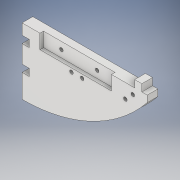
# Autodesk Inventor part: CP003
Saved by Autodesk Inventor 2017 SP1 (Build 210196100, 196)
## iProperties
Created: 2017-05-15
Part Number: CP003
Material: ABS Plastic
Document SubType Name: Modeling
Designer: zallen
Density: 1.06 g/cm^3
Appearance: Smooth - White
Mass: 174.081 g
Surface Area: 322.497 cm^2
Volume: 164.227 cm^3
Author: zallen
Autodesk Inventor part; units mm, degrees
ref_plane "YZ Plane" through (0, 0, 0) normal (1, 0, 0) x (0, 1, 0)
ref_plane "XZ Plane" through (0, 0, 0) normal (0, 1, 0) x (-1, 0, 0)
ref_plane "XY Plane" through (0, 0, 0) normal (0, 0, 1) x (1, 0, 0)
sketch "Sketch1" plane through (0, 0, 0) normal (0, 0, 1) x (1, 0, 0)
  circle A0 centre (0, 132.2876) radius 225 construction
  circle A1 centre (0, 132.2876) radius 200 construction
  line L0 (150, 132.2876) -> (150, 0) construction
  line L1 (150, 0) -> (0, 0)
  line L2 (0, 0) -> (0, -92.7124)
  arc A2 (0, -92.7124) -> (175, -9.1338) centre (0, 132.2876) ccw
  line L3 (157.5, 0) -> (157.5, 10)
  line L4 (157.5, 10) -> (167.5, 10)
  line L5 (167.5, 10) -> (167.5, 0)
  line L6 (150, 0) -> (157.5, 0)
  line L7 (175, -35.9935) -> (175, -9.1338) construction
  line L8 (175, 0) -> (175, -9.1338)
  line L9 (167.5, 0) -> (175, 0)
  line L10 (0, 132.2876) -> (0, -92.7124) construction
  line L11 (0, 132.2876) -> (225, 132.2876) construction
  line L12 (0, 0) -> (130.6185, 0) construction
  dimension "d0" = 450
  dimension "d1" = 25
  dimension "d3" = 10
  dimension "d4" = 10
  dimension "d6" = 7.5
  dimension "d7" = 90
  dimension "d9" = 25
  dimension "d12" = 90
  dimension "d13" = 75
  dimension "d14" = 90
  constraints: 26 end point, 6 point on circle, 5 point on line, 4 perpendicular, 3 horizontal, 2 centre point, 1 coincident, 1 collinear, 1 concentric, 1 parallel, 3 other
  measures "d0" diameter of A0
  measures "d3" distance of L3.start L3.end
  measures "d4" distance of L3.end L4.end
  measures "d6" distance of L0.end L3.start
  measures "d7" angle of L5 L4
  measures "d9" distance between parallel lines of L7 L0
  measures "d12" angle of L10 L11
  measures "d13" distance of L11.end L0.start
  measures "d14" angle of L1 L0
extrude "Extrusion1" add sketch "Sketch1" along normal blind 15
sketch "Sketch2" plane through (0, 0, 15) normal (0, 0, 1) x (1, 0, 0)
  line L0 (0, 0) -> (0, -92.7124) projected
  line L1 (0, -15) -> (10, -15)
  line L2 (10, -15) -> (10, -25)
  line L3 (10, -25) -> (0, -25)
  line L4 (0, -25) -> (0, -15)
  line L5 (0, -50) -> (10, -50)
  line L6 (10, -50) -> (10, -60)
  line L7 (10, -60) -> (0, -60)
  line L8 (0, -60) -> (0, -50)
  line L9 (157.5, 0) -> (0, 0) projected
  dimension "d15" = 10
  dimension "d16" = 10
  dimension "d17" = 10
  dimension "d18" = 10
  dimension "d19" = 25
  dimension "d20" = 15
  constraints: 16 end point, 4 parallel, 2 horizontal, 2 perpendicular, 2 point on line
  measures "d15" distance of L2.end L3.end
  measures "d16" distance of L1.end L2.end
  measures "d17" distance of L6.end L7.end
  measures "d18" distance of L5.end L6.end
  measures "d19" distance between parallel lines of L5 L3
  measures "d20" distance between parallel lines of L1 L9
extrude "Extrusion2" cut sketch "Sketch2" against normal blind 15
sketch "Sketch3" plane through (0, 0, 15) normal (0, 0, 1) x (1, 0, 0)
  line L0 (157.5, 0) -> (0, 0) construction
  line L1 (25, 0) -> (125, 0) construction
  line L2 (125, 0) -> (125, -20) construction
  line L3 (125, -20) -> (25, -20) construction
  line L4 (25, -20) -> (25, 0) construction
  circle A0 centre (50, -10) radius 2.5
  circle A1 centre (100, -10) radius 2.5
  dimension "d23" = 100
  dimension "d24" = 20
  dimension "d25" = 25
  dimension "d26" = 5
  dimension "d27" = 5
  dimension "d28" = 25
  dimension "d29" = 25
  constraints: 8 end point, 2 centre point, 2 parallel, 1 horizontal, 1 perpendicular, 1 point on line
  measures "d23" distance of L2.end L3.end
  measures "d24" distance of L1.end L2.end
  measures "d25" distance from line of L0.end L4
  measures "d26" diameter of A0
  measures "d27" diameter of A1
  measures "d28" distance from line of L4 A0.centre
  measures "d29" distance from line of L2 A1.centre
extrude "Extrusion3" cut sketch "Sketch3" against normal through all
thread "Thread1" size "M5x0.8" class "6H" standard "ANSI Metric M Profile" full length
thread "Thread2" size "M5x0.8" class "6H" standard "ANSI Metric M Profile" full length
sketch "Sketch4" plane through (0, 0, 15) normal (0, 0, 1) x (1, 0, 0)
  line L0 (157.5, 0) -> (0, 0) projected
  line L1 (25, 0) -> (125, 0)
  line L2 (125, 0) -> (125, -20)
  line L3 (125, -20) -> (25, -20)
  line L4 (25, -20) -> (25, 0)
  dimension "d36" = 100
  dimension "d37" = 20
  dimension "d38" = 25
  constraints: 8 end point, 2 parallel, 1 horizontal, 1 perpendicular, 1 point on line
  measures "d36" distance of L2.end L3.end
  measures "d37" distance of L1.end L2.end
  measures "d38" distance from line of L0.end L4
extrude "Extrusion4" cut sketch "Sketch4" against normal blind 5
sketch "Sketch5" plane through (0, 0, 15) normal (0, 0, 1) x (1, 0, 0)
  circle A0 centre (0, 132.2876) radius 225 construction
  arc A1 (0, -92.7124) -> (175, -9.1338) centre (0, 132.2876) ccw construction
  circle A2 centre (0, 132.2876) radius 210 construction
  circle A3 centre (144.4906, -20.1016) radius 2.5
  circle A4 centre (155, -9.3987) radius 2.5
  line L0 (175, -9.1338) -> (175, 0) projected
  point P0 (0, 0)
  dimension "d41" = 450
  dimension "d42" = 15
  dimension "d43" = 5
  dimension "d44" = 5
  dimension "d45" = 15
  dimension "d46" = 20
  constraints: 4 centre point, 2 point on circle, 1 concentric
  measures "d41" diameter of A0
  measures "d42" radial gap between concentric circles of A0 A2
  measures "d43" diameter of A3
  measures "d44" diameter of A4
  measures "d45" distance of A4.centre A3.centre
  measures "d46" distance from line of L0 A4.centre
extrude "Extrusion5" cut sketch "Sketch5" against normal through all
thread "Thread3" size "M5x0.8" class "6H" standard "ANSI Metric M Profile" full length
thread "Thread4" size "M5x0.8" class "6H" standard "ANSI Metric M Profile" full length
sketch "Sketch6" plane through (0, 0, 15) normal (0, 0, 1) x (1, 0, 0)
  circle A0 centre (69.0912, -25.1338) radius 2.5
  circle A1 centre (84.0912, -25.1338) radius 2.5
  line L0 (25, 0) -> (125, 0) projected
  arc A2 (0, -92.7124) -> (175, -9.1338) centre (0, 132.2876) ccw construction
  line L1 (175, -9.1338) -> (-10.7224, -9.1338) construction
  line L2 (0, 0) -> (0, -15) construction
  dimension "d53" = 5
  dimension "d54" = 5
  dimension "d56" = 16
  dimension "d57" = 69.0912
  dimension "d58" = 15
  constraints: 2 centre point, 2 end point, 1 horizontal alignment, 1 perpendicular
  measures "d53" diameter of A0
  measures "d54" diameter of A1
  measures "d56" distance from line of A0.centre L1
  measures "d57" distance from line of L2 A0.centre
  measures "d58" distance of A1.centre A0.centre
extrude "Extrusion6" cut sketch "Sketch6" against normal through all
thread "Thread5" size "M5x0.8" class "6H" standard "ANSI Metric M Profile" full length
thread "Thread6" size "M5x0.8" class "6H" standard "ANSI Metric M Profile" full length
body "Solid1"
